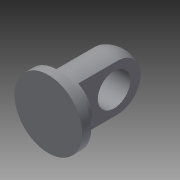
# Autodesk Inventor part: pruzinauvhyt
Saved by Autodesk Inventor 2013 (Build 170138000, 138)
## iProperties
Created: 2015-06-12
Part Number: pruzinauvhyt
Material: Generic
Document SubType Name: Modeling
Designer: Jufo
Density: 1 g/cm^3
Author: Jufo
Autodesk Inventor part; units mm, degrees
ref_plane "YZ Plane" through (0, 0, 0) normal (1, 0, 0) x (0, 1, 0)
ref_plane "XZ Plane" through (0, 0, 0) normal (0, 1, 0) x (-1, 0, 0)
ref_plane "XY Plane" through (0, 0, 0) normal (0, 0, 1) x (1, 0, 0)
sketch "Sketch1" plane through (0, 0, 0) normal (0, 1, 0) x (-1, 0, 0)
  circle A0 centre (0, 0) radius 5.2
  dimension "d0" = 10.4
  constraints: 1 centre point, 1 coincident
  measures "d0" diameter of A0
extrude "Extrusion1" add sketch "Sketch1" along normal blind 1.4
sketch "Sketch2" plane through (0, 1.4, 0) normal (0, 1, 0) x (1, 0, 0)
  circle A0 centre (0, 0) radius 5.2 projected
  circle A1 centre (0, 0) radius 4
  dimension "d3" = 8
  constraints: 1 centre point, 1 coincident
  measures "d3" diameter of A1
extrude "Extrusion2" add sketch "Sketch2" along normal blind 1.4 contours A1
sketch "Sketch3" plane through (0, 2.8, 0) normal (0, 1, 0) x (1, 0, 0)
  circle A0 centre (0, 0) radius 4 projected
  line L0 (-1.8, 3.5721) -> (-1.8, -3.5721)
  line L1 (1.8, 3.5721) -> (1.8, -3.5721)
  arc A1 (-1.8, -3.5721) -> (1.8, -3.5721) centre (0, 0) ccw
  arc A2 (1.8, 3.5721) -> (-1.8, 3.5721) centre (0, 0) ccw
  constraints: 6 point on circle, 4 end point, 2 centre point, 2 concentric
extrude "Extrusion3" add sketch "Sketch3" along normal blind 10 contours L1 A0 L0
sketch "Sketch4" plane through (1.8, 2.8, 3.5721) normal (1, 0, 0) x (0, 0, -1)
  line L0 (0, 10) -> (7.1442, 10) projected
  line L1 (0, 0) -> (0, 10) projected
  line L2 (3.5721, 10) -> (3.5721, 5.5)
  circle A0 centre (3.5721, 5.5) radius 2.5
  point P0 (3.5721, -2.8)
  dimension "d9" = 4.5
  dimension "d10" = 5
  constraints: 2 end point, 1 centre point, 1 coincident, 1 midpoint, 1 parallel
  measures "d9" distance of L2.start L2.end
  measures "d10" diameter of A0
extrude "Extrusion4" cut sketch "Sketch4" against normal blind 10
fillet "Fillet1" radius 4 2 edges at (0, 12.8, 4) (0, 12.8, -4)
body "Solid1"
